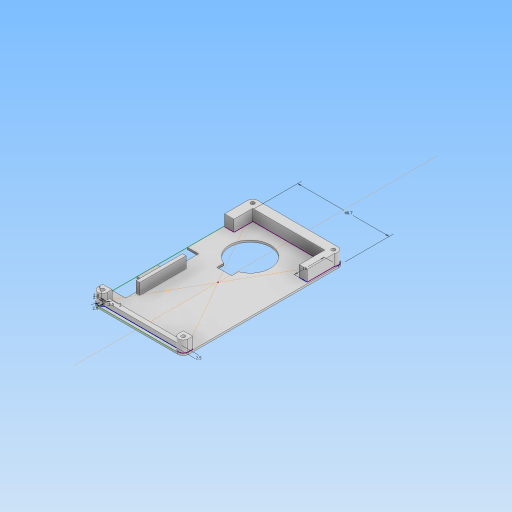
# Autodesk Inventor part: my_back_metric
Saved by Autodesk Inventor 2023 (Build 270158000, 158)
## iProperties
Created: 2023-04-17
Part Number: my_back_metric
Material: Generic
Document SubType Name: Modeling
Designer: kar
Density: 1 g/cm^3
Appearance: Default
Author: kar
Autodesk Inventor part; units mm, degrees
ref_plane "YZ Plane" through (0, 0, 0) normal (1, 0, 0) x (0, 1, 0)
ref_plane "XZ Plane" through (0, 0, 0) normal (0, 1, 0) x (-1, 0, 0)
ref_plane "XY Plane" through (0, 0, 0) normal (0, 0, 1) x (1, 0, 0)
sketch "Sketch1" plane through (0, 0, 0) normal (0, 1, 0) x (-1, 0, 0)
  line L0 (-21.35, 42.8) -> (21.35, 42.8)
  line L1 (24.35, 39.8) -> (24.35, -39.8)
  line L2 (21.35, -42.8) -> (-21.35, -42.8)
  line L3 (-24.35, -39.8) -> (-24.35, 39.8)
  arc A0 (24.35, 39.8) -> (21.35, 42.8) centre (21.35, 39.8) ccw
  arc A1 (21.35, -42.8) -> (24.35, -39.8) centre (21.35, -39.8) ccw
  arc A2 (-24.35, -39.8) -> (-21.35, -42.8) centre (-21.35, -39.8) ccw
  arc A3 (-21.35, 42.8) -> (-24.35, 39.8) centre (-21.35, 39.8) ccw
  line L4 (-47.6975, 0) -> (69.2667, 0) construction
  point P0 (0, 0)
  dimension "d2" = 3
  constraints: 10 end point, 8 point on circle, 8 tangent, 4 centre point, 3 equal radius, 2 horizontal, 2 parallel, 1 perpendicular
  measures "d2" radius of A0
sketch "Sketch2" plane through (0, 0, 0) normal (0, 1, 0) x (-1, 0, 0)
  line L0 (-24.35, 42.8) -> (24.35, -42.8) construction
  line L1 (24.35, 42.8) -> (-24.35, -42.8) construction
  circle A0 centre (21.45, 39.9) radius 1
  line L2 (0, 76.772) -> (0, -116.4578) construction
  circle A1 centre (21.45, 39.9) radius 2.5
  line L3 (19.2849, 41.15) -> (-19.2849, 41.15)
  line L4 (-19.2849, 41.15) -> (-19.2849, 38.65)
  line L5 (-19.2849, 38.65) -> (19.2849, 38.65)
  line L6 (19.2849, 38.65) -> (19.2849, 41.15)
  circle A2 centre (-21.45, 39.9) radius 2.5
  circle A3 centre (-21.45, 39.9) radius 1
  line L7 (23.95, 39.9) -> (18.95, 39.9)
  line L8 (18.95, 39.9) -> (18.95, 37.4)
  line L9 (18.95, 37.4) -> (23.95, 37.4)
  line L10 (-23.95, 39.9) -> (-18.95, 39.9)
  line L11 (-18.95, 37.4) -> (-23.95, 37.4)
  line L12 (-18.95, 39.9) -> (-18.95, 37.4)
  line L13 (24.35, 39.8) -> (24.35, -39.8) projected
  line L14 (-21.35, 42.8) -> (21.35, 42.8) projected
  arc A4 (24.35, 39.8) -> (21.35, 42.8) centre (21.35, 39.8) ccw projected
  line L15 (23.95, 39.9) -> (23.95, 37.4)
  line L16 (-23.95, 37.4) -> (-23.95, 39.9)
  point P0 (0, 0)
  point P1 (0, 0)
  point P2 (-21.35, 39.8)
  point P3 (21.45, 39.9)
  point P4 (-18.95, 38.65)
  point P5 (18.95, 38.65)
  point P6 (-21.45, 37.4)
  dimension "d16" = 48.7
  dimension "d17" = 2
  dimension "d18" = 5
  dimension "d19" = 2.5
  dimension "d20" = 2.5
  dimension "d23" = 2.9
  dimension "d24" = 2.9
  dimension "d25" = 2.9
  constraints: 30 end point, 6 symmetric about line, 4 vertical, 3 centre point, 3 midpoint, 3 parallel, 3 point on circle, 2 coincident, 2 horizontal, 2 perpendicular, 1 tangent, 5 other
  measures "d16" distance of L0.end L1.end
  measures "d17" diameter of A0
  measures "d18" diameter of A1
  measures "d19" distance between parallel lines of L5 L3
  measures "d20" distance of L8.start L8.end
  measures "d23" distance from line of L13 point (21.45, 39.9)
  measures "d24" distance from line of L14 A0.centre
  measures "d25" distance from line of L13 A0.centre
sketch "Sketch4" plane through (0, 0, 0) normal (0, 1, 0) x (-1, 0, 0)
  circle A0 centre (21.45, -39.9) radius 2.5
  circle A1 centre (21.45, -39.9) radius 1
  circle A2 centre (-21.45, -39.9) radius 1
  circle A3 centre (-21.45, -39.9) radius 2.5
  line L0 (23.95, -39.9) -> (18.95, -39.9)
  line L1 (18.95, -39.9) -> (18.95, -27.4467)
  line L2 (18.95, -27.4467) -> (23.95, -27.4467)
  line L3 (23.95, -27.4467) -> (23.95, -39.9)
  line L4 (21.45, -37.4) -> (-21.45, -37.4)
  line L5 (-21.45, -37.4) -> (-21.45, -42.4)
  line L6 (-21.45, -42.4) -> (21.45, -42.4)
  line L7 (21.45, -42.4) -> (21.45, -37.4)
  line L8 (-19.377, -38.5026) -> (-23.523, -38.5026)
  line L9 (-23.523, -38.5026) -> (-23.523, -23.9)
  line L10 (-23.523, -23.9) -> (-19.377, -23.9)
  line L11 (-19.377, -23.9) -> (-19.377, -38.5026)
  point P0 (0, 0)
  point P1 (21.35, -42.8)
  point P2 (24.35, -39.8)
  point P3 (21.35, -39.8)
  point P4 (-24.35, -39.8)
  point P5 (-21.35, -42.8)
  point P6 (-21.35, -39.8)
  point P7 (18.95, -37.4)
  point P8 (-19.377, -37.4)
  point P9 (-21.45, -23.9)
  point P10 (-21.45, -39.9)
  dimension "d52" = 16
  constraints: 24 end point, 6 parallel, 5 point on circle, 4 centre point, 3 horizontal, 3 perpendicular, 2 coincident, 2 midpoint, 1 other
  measures "d52" distance from line of L10 A3.centre
sketch "Sketch5" plane through (0, 0, 0) normal (0, 1, 0) x (-1, 0, 0)
  line L0 (24.35, 39.8) -> (24.35, -39.8) projected
  line L1 (24.35, 8) -> (18.35, 8)
  line L2 (18.35, 8) -> (18.35, -8)
  line L3 (18.35, -8) -> (24.35, -8)
  line L4 (24.35, -8) -> (24.35, 8)
  line L5 (31.157, 0) -> (-16.4919, 0) projected
  point P0 (0, 0)
  point P1 (18.35, 0)
  point P2 (21.35, -8)
  dimension "d21" = 16
  dimension "d22" = 6
  constraints: 8 end point, 2 midpoint, 2 parallel, 2 point on line, 1 horizontal, 1 perpendicular
  measures "d21" distance from line of point (21.35, -8) L1
  measures "d22" distance of L2.end L3.end
extrude "Extrusion2" add sketch "Sketch1" against normal blind 1
extrude "Extrusion3" add sketch "Sketch2" along normal blind 2.5 contours A1 L8 L5 L12 A2 L3
extrude "Extrusion4" add sketch "Sketch2" along normal blind 5.9 contours L7 A1 L6 A0 | A0 L7 L6 A1 | L15 L9 A1 | L7 A1 L6 | L6 A1 L7 | L9 L8 L5 A1 | L5 L8 A1 | A2 L10 L4 | L4 L10 A3 A2 | L10 A2 L4 | L4 A2 L10 A3 | L12 L5 A2 | A2 L11 L16 | L12 L11 A2 L5
extrude "Extrusion5" add sketch "Sketch4" along normal up to surface (5.9 mm away) contours L0 A1 L7 A0 | A0 L7 A1 L0 | A0 L4 L1 L2 L3 | L7 A1 L0 A0 | A0 L1 L4 | L6 A3 L11 L4 L1 A0 | A0 L0 A1 L7 | L5 A2 L8 A3 | A3 L8 L5 A2 | L11 A3 L4 | L4 A3 L9 L10 L11 | A3 L5 L8 | A3 L8 L5
extrude "Extrusion6" cut sketch "Sketch4" along normal through all both and the other way through all contours L0 L7 A1 | A1 L7 L0 | L7 L0 A1 | A1 L0 L7 | L5 A2 | A2 L5
extrude "Extrusion7" cut sketch "Sketch2" along normal through all both and the other way through all contours L7 A0 | A0 L7 | L10 A3 | A3 L10
extrude "Extrusion8" cut sketch "Sketch5" along normal through all both and the other way through all
sketch "Sketch6" plane through (0, -1, 0) normal (0, -1, 0) x (1, 0, 0)
  arc A0 (5.4227, -14.164) -> (0.5528, -10.3702) centre (-3.3726, -20.4316) ccw
  line L0 (0.5528, -10.3702) -> (0.5528, -6.679)
  line L1 (0.5528, -6.679) -> (-2.7471, -6.679)
  line L2 (-2.7471, -6.679) -> (-3.9471, -6.679)
  line L3 (-3.9471, -6.679) -> (-7.1971, -6.679)
  line L4 (-7.1971, -6.679) -> (-7.1971, -10.3315)
  arc A1 (-7.1971, -10.3315) -> (-12.1679, -14.164) centre (-3.3726, -20.4316) ccw
  arc A2 (-12.45, -14.5801) -> (-13.3806, -16.3723) centre (-3.3726, -20.4316) ccw
  arc A3 (-13.4465, -16.5387) -> (-13.4465, -24.3246) centre (-3.3726, -20.4316) ccw
  arc A4 (-13.3806, -24.491) -> (-12.45, -26.2832) centre (-3.3726, -20.4316) ccw
  arc A5 (-12.1679, -26.6992) -> (5.4227, -26.6992) centre (-3.3726, -20.4316) ccw
  arc A6 (5.7048, -26.2832) -> (6.6355, -24.491) centre (-3.3726, -20.4316) ccw
  arc A7 (6.7014, -24.3246) -> (6.7014, -16.5387) centre (-3.3726, -20.4316) ccw
  arc A8 (6.6355, -16.3723) -> (5.7048, -14.5801) centre (-3.3726, -20.4316) ccw
  arc A9 (-7.1971, -10.3315) -> (0.5528, -10.3702) centre (-3.3726, -20.4316) ccw
  point P0 (0, 0)
  point P1 (-13.3806, -24.491)
  point P2 (-12.45, -26.2832)
  point P3 (-12.1679, -26.6992)
  point P4 (5.7048, -26.2832)
  point P5 (6.6355, -24.491)
  point P6 (6.7014, -24.3246)
  point P7 (6.6355, -16.3723)
  point P8 (5.7048, -14.5801)
  point P9 (5.4227, -14.164)
  constraints: 20 point on circle, 10 centre point, 10 end point, 1 coincident, 1 concentric
extrude "Extrusion9" cut sketch "Sketch6" along normal through all both and the other way through all
sketch "Sketch7" plane through (0, -1, 0) normal (0, -1, 0) x (1, 0, 0)
  line L0 (-9.9467, 38.1508) -> (9.6849, 38.1508) construction
  line L1 (9.6849, 38.1508) -> (9.6849, 29.6438) construction
  line L2 (9.6849, 29.6438) -> (-9.9467, 29.6438) construction
  line L3 (-9.9467, 29.6438) -> (-9.9467, 38.1508) construction
  point P0 (0, 0)
  constraints: 2 other
sketch "Sketch8" plane through (0, -1, 0) normal (0, -1, 0) x (1, 0, 0)
  line L0 (-24.35, 39.8) -> (-24.35, -39.8) projected
  line L1 (-24.35, 8) -> (-24.35, 39.8) projected
  line L2 (-24.35, 18.8) -> (-17.35, 18.8)
  line L3 (-17.35, 18.8) -> (-17.35, 31.8)
  line L4 (-17.35, 31.8) -> (-24.35, 31.8)
  line L5 (-24.35, 31.8) -> (-24.35, 18.8)
  line L6 (21.35, 42.8) -> (-21.35, 42.8) projected
  point P0 (0, 0)
  dimension "d43" = 7
  dimension "d45" = 24
  dimension "d46" = 11
  constraints: 8 end point, 2 parallel, 1 horizontal, 1 perpendicular, 1 point on line
  measures "d43" distance of L4.end L3.end
  measures "d45" distance between parallel lines of L6 L2
  measures "d46" distance between parallel lines of L6 L4
extrude "Extrusion10" cut sketch "Sketch8" along normal through all both and the other way through all
sketch "Sketch9" plane through (0, 0, 0) normal (0, 1, 0) x (1, 0, 0)
  line L0 (-14.8468, -26.7931) -> (-16.7148, -26.7931)
  line L1 (-16.7148, -26.7931) -> (-16.7148, -2.0705)
  line L2 (-16.7148, -2.0705) -> (-14.8468, -2.0705)
  line L3 (-14.8468, -2.0705) -> (-14.8468, -26.7931)
  point P0 (0, 0)
  constraints: 8 end point, 2 parallel, 1 horizontal, 1 perpendicular
extrude "Extrusion11" add sketch "Sketch9" along normal up to surface (5.9 mm away)
body "Solid2"
